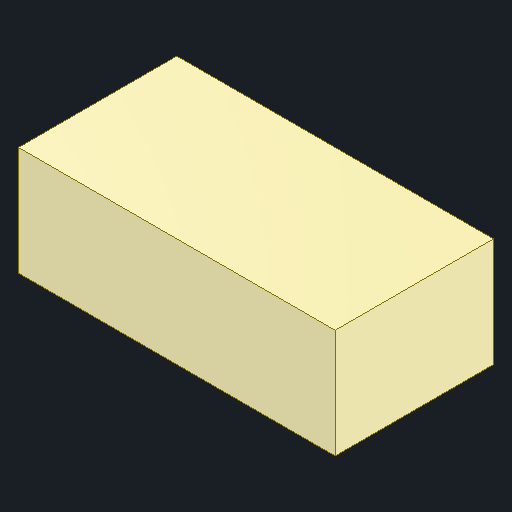
# Autodesk Inventor part: Small light
Saved by Autodesk Inventor 2026.2 (Build 302298010, 298A)
## iProperties
Created: 2026-03-31
Part Number: Small light
Material: Nylon 6/6
Document SubType Name: Modeling
Designer: piete
Density: 1.13 g/cm^3
Appearance: Nylon 6
Author: piete
Autodesk Inventor part; units mm, degrees
ref_plane "YZ Plane" through (0, 0, 0) normal (1, 0, 0) x (0, 1, 0)
ref_plane "XZ Plane" through (0, 0, 0) normal (0, 1, 0) x (-1, 0, 0)
ref_plane "XY Plane" through (0, 0, 0) normal (0, 0, 1) x (1, 0, 0)
sketch "Sketch1" plane through (0, 0, 0) normal (0, 1, 0) x (-1, 0, 0)
  line L0 (0.8, 0.4) -> (-0.8, 0.4)
  line L1 (-0.8, 0.4) -> (-0.8, -0.4)
  line L2 (-0.8, -0.4) -> (0.8, -0.4)
  line L3 (0.8, -0.4) -> (0.8, 0.4)
  point P0 (0, 0)
  dimension "d0" = 1.6
  dimension "d1" = 0.8
  dimension "d2" = 0.8
  dimension "d3" = 0.4
  constraints: 8 end point, 2 parallel, 1 horizontal, 1 perpendicular
  measures "d0" distance of L2.end L1.end
  measures "d1" distance of L1.end L0.end
  measures "d2" distance from line of point (0, 0) L3
  measures "d3" distance from line of point (0, 0) L0
extrude "Extrusion1" add sketch "Sketch1" along normal blind 0.55
equation "\"d2\" = 0.5 * d0"
equation "\"d3\" = 0.5 * d1"
body "Solid1"
